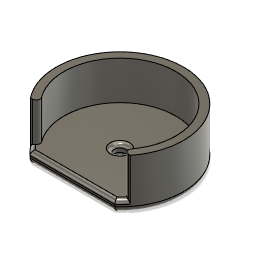
Motor cover v1 (Autodesk Fusion 360 design; units mm, degrees)
Autodesk Fusion 360 part; units mm, degrees
sketch "Sketch1" plane through (0, 0, 0) normal (0, 1, 0) x (1, 0, 0)
  line L0 (-11, -12.2984) -> (11, -12.2984)
  arc A0 (11, -12.2984) -> (-11, -12.2984) centre (0, 0) ccw
  dimension "d1" = 33
  constraint coincident A0.centre origin
  measures "d1" diameter of A0
extrude "Extrude1" add sketch "Sketch1" along normal blind 3
sketch "Sketch2" plane through (0, 3, 0) normal (0, 1, 0) x (-1, 0, 0)
  arc A0 (-11, 12.2984) -> (11, 12.2984) centre (0, 0) ccw
  line L0 (11, 12.2984) -> (-11, 12.2984)
  arc A1 (-10.2553, 10.2508) -> (10.2075, 10.2984) centre (0, 0) ccw
  arc A2 (-12.9295, 10.2508) -> (12.8916, 10.2984) centre (0, 0) ccw
  line L1 (10.2075, 10.2984) -> (12.8916, 10.2984)
  line L2 (-10.2553, 10.2508) -> (-12.9295, 10.2508)
  constraint concentric A0 A1
  constraint horizontal L1
  constraint parallel L0 L2
extrude "Extrude2" add sketch "Sketch2" along normal blind 10 contours A0 A1 A2 L1 L2
sketch "Sketch3" plane through (0, 3, 0) normal (0, 1, 0) x (-1, 0, 0)
  line L0 (-12.9295, 10.2508) -> (-10.2553, 10.2508)
  arc A0 (-10.2553, 10.2508) -> (10.2075, 10.2984) centre (0, 0) ccw
  line L1 (10.2075, 10.2984) -> (12.8916, 10.2984)
  arc A1 (12.8916, 10.2984) -> (11, 12.2984) centre (0, 0) ccw
  line L2 (11, 12.2984) -> (-11, 12.2984)
  arc A2 (-11, 12.2984) -> (-12.9295, 10.2508) centre (0, 0) ccw
  circle A3 centre (0, 0) radius 1.5
  dimension "d8" = 3
  constraint coincident A0.centre A1.centre
  measures "d8" diameter of A3
extrude "Extrude3" cut sketch "Sketch3" against normal blind 10 contours A3
fillet "Fillet1" radius 1 2 edges at (-10.2075, 8, 10.2984) (10.2553, 8, 10.2508)
fillet "Fillet2" radius 1.5 2 edges at (0, 0, -16.5) (0, 0, 12.2984)
fillet "Fillet3" radius 1 1 edges at (1.3985, 0, -0.5424)
fillet "Fillet4" radius 1 1 edges at (1.3985, 3, 0.5424)
fillet "Fillet5" radius 1 3 edges at (-11.9876, 3, 11.3379) (0, 3, 12.2984) (12.0085, 3, 11.3158)
